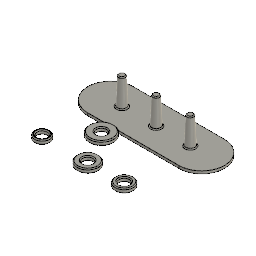
Towers_of_Hanoi (Autodesk Fusion 360 design; units mm, degrees)
Autodesk Fusion 360 part; units mm, degrees
sketch "Sketch1" plane through (0, 0, 0) normal (0, 0, 1) x (1, 0, 0)
  line L0 (0, 0) -> (100, 0)
  line L1 (100, 0) -> (100, 50)
  line L2 (100, 50) -> (0, 50)
  line L3 (0, 50) -> (0, 0)
  arc A0 (100, 0) -> (100, 50) centre (100, 25) ccw
  arc A1 (0, 50) -> (0, 0) centre (0, 25) ccw
  line L4 (0, 25) -> (100, 25) construction
  circle A2 centre (12.5, 25) radius 5
  line L5 (50, 0) -> (50, 50) construction
  circle A3 centre (50, 25) radius 5
  circle A4 centre (87.5, 25) radius 5
  dimension "d3" = 100
  dimension "d4" = 50
  dimension "d6" = 10
  dimension "d7" = 10
  dimension "d8" = 10
  dimension "d9" = 37.5
  dimension "d10" = 37.5
  constraint horizontal L0
  constraint vertical L1
  constraint horizontal L2
  constraint vertical L3
  constraint coincident L0.start L3.end
  constraint tangent L0 A0
  constraint coincident A1.centre L4.start
  constraint coincident A0.centre L4.end
  constraint coincident L4 A2.centre
  constraint midpoint L0 L5.start
  constraint midpoint L2 L5.end
  constraint midpoint L5 A3.centre
  constraint coincident L4 A4.centre
  measures "d3" distance of L0.start L0.end
  measures "d4" distance of L0.start L2.end
  measures "d6" diameter of A2
  measures "d7" diameter of A3
  measures "d8" diameter of A4
  measures "d9" distance of A3.centre A4.centre
  measures "d10" distance of A2.centre A3.centre
extrude "Extrude1" add sketch "Sketch1" against normal blind 3 contours L0 L1 L2 L3 | L3 A1 | L1 A0 | A2 | A3 | A4 makes body 1
extrude "Extrude2" add sketch "Sketch1" along normal blind 30 draft -2.5 contours A2 | A3 | A4 bodies 1
sketch "Sketch2" plane through (0, 0, 0) normal (0, 0, 1) x (1, 0, 0)
  circle A0 centre (0, -50) radius 8.3335
  circle A1 centre (0, -50) radius 5.5
  circle A2 centre (50, -50) radius 11.6665
  circle A3 centre (50, -50) radius 5.5
  circle A4 centre (90, -50) radius 10
  circle A5 centre (90, -50) radius 5.5
  circle A6 centre (30, -15) radius 13.3335
  circle A7 centre (30, -15) radius 5.5
  dimension "d17" = 16.667
  dimension "d18" = 11
  dimension "d20" = 23.333
  dimension "d21" = 11
  dimension "d22" = 20
  dimension "d23" = 11
  dimension "d28" = 26.667
  dimension "d29" = 11
  constraint concentric A0 A1
  constraint concentric A2 A3
  constraint concentric A4 A5
  constraint concentric A6 A7
  measures "d17" diameter of A0
  measures "d18" diameter of A1
  measures "d20" diameter of A2
  measures "d21" diameter of A3
  measures "d22" diameter of A4
  measures "d23" diameter of A5
  measures "d28" diameter of A6
  measures "d29" diameter of A7
extrude "Extrude3" add sketch "Sketch2" along normal blind 5 separate body makes body 2 at (8.3231, -50.4154, 3.3333) makes body 3 at (61.652, -50.5815, 3.3333) makes body 4 at (99.9876, -50.4985, 3.3333) makes body 5 at (40.6727, -15.6624, 0)
fillet "Fillet1" radius 1 3 edges at (82.8384, 26.8081, 0) (45.3384, 26.8081, 0) (7.8384, 26.8081, 0) on bodies 1
fillet "Fillet2" radius 1 3 edges at (84.0596, 26.3344, 30) (46.5596, 26.3344, 30) (9.0596, 26.3344, 30) on bodies 1
chamfer "Chamfer1" distance 1 angle 45 16 edges at (39.123, -54.2188, 0) (44.8722, -48.0111, 0) (39.123, -54.2188, 5) (44.8722, -48.0111, 5) (80.6767, -53.6162, 0) (84.8722, -48.0111, 0) (80.6767, -53.6162, 5) (84.8722, -48.0111, 5) (-7.7695, -53.0135, 0) (-5.1278, -48.0111, 0) (-7.7695, -53.0135, 5) (-5.1278, -48.0111, 5) (17.5688, -19.8216, 0) (24.8722, -13.0111, 0) (17.5688, -19.8216, 5) (24.8722, -13.0111, 5) on bodies 2 3 4 5
equation "baseLength = 100 mm"
equation "baseWidth = 50 mm"
equation "d3 = baseLength"
equation "d4 = baseWidth"
equation "pegBaseDiameter = 10 mm"
equation "d6 = pegBaseDiameter"
equation "d7 = pegBaseDiameter"
equation "d8 = pegBaseDiameter"
equation "d9 = ( baseLength + baseWidth ) / 4"
equation "d10 = ( baseLength + baseWidth ) / 4"
equation "baseThickness = 3 mm"
equation "d12 = -baseThickness"
equation "pegHeight = 30 mm"
equation "d15 = pegHeight"
equation "d18 = pegBaseDiameter + 1 mm"
equation "diskThickness = 5 mm"
equation "d21 = pegBaseDiameter + 1 mm"
equation "d23 = pegBaseDiameter + 1 mm"
equation "d24 = diskThickness"
equation "d29 = pegBaseDiameter + 1 mm"
named bodies: "Base"
